Picture Hanger (Autodesk Fusion 360 design; units mm, degrees)
Autodesk Fusion 360 part; units mm, degrees
note: some values were not read from the file. Set by a fixed rule: which sketch regions a step uses.
sketch "Sketch1" plane through (0, 0, 0) normal (0, 0, 1) x (1, 0, 0)
  circle A0 centre (0, 0) radius 7.5
  circle A1 centre (0, 0) radius 6
  circle A2 centre (0, 0) radius 4
  line L0 (-12, 0) -> (12, 0)
  line L1 (12, 0) -> (12, 11)
  line L2 (12, 11) -> (-12, 11)
  line L3 (-12, 11) -> (-12, 0)
  circle A3 centre (0, 0) radius 2.5
  dimension "d1" = 15
  dimension "d2" = 12
  dimension "d3" = 8
  dimension "d12" = 5
  constraint coincident A0.centre A1.centre
  constraint concentric A0 A1
  constraint horizontal L0
  constraint vertical L1
  constraint horizontal L2
  constraint vertical L3
  constraint concentric A1 A3
  measures "d1" diameter of A0
  measures "d2" diameter of A1
  measures "d3" diameter of A2
  measures "d12" diameter of A3
extrude "Extrude1" add sketch "Sketch1" along normal blind 2 contours A0 A1 L0 | A0 A1 L0 | A1 A2 L0 | A1 A2 L0 | A2 L0 A3 | A2 L0 A3
extrude "Extrude2" add sketch "Sketch1" along normal blind 12 contours A0 A1 L0 | A0 A1 L0
extrude "Extrude3" add sketch "Sketch1" along normal blind 3 from surface at 9 contours A1 A2 L0 picked at (-4.096, 3.3939)
fillet "Fillet1" radius 2 1 edges at (0, 6, 9)
